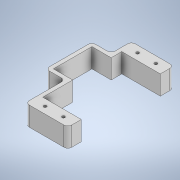
# Autodesk Inventor part: servo_bracket
Saved by Autodesk Inventor 2020 (Build 240168000, 168)
## iProperties
Created: 2019-05-08
Part Number: servo_bracket
Material: Generic
Document SubType Name: Modeling
Designer: erwin
Density: 1 g/cm^3
Appearance: Default
Author: erwin
Autodesk Inventor part; units mm, degrees
ref_plane "YZ Plane" through (0, 0, 0) normal (1, 0, 0) x (0, 1, 0)
ref_plane "XZ Plane" through (0, 0, 0) normal (0, 1, 0) x (-1, 0, 0)
ref_plane "XY Plane" through (0, 0, 0) normal (0, 0, 1) x (1, 0, 0)
sketch "Sketch1" plane through (0, 0, 0) normal (0, 1, 0) x (-1, 0, 0)
  line L0 (-9.6397, 29.7296) -> (10.3603, 29.7296)
  line L1 (12.3603, 29.7296) -> (12.3603, 36.7296)
  line L2 (12.3603, 36.7296) -> (-9.6397, 36.7296)
  line L3 (-9.6397, 36.7296) -> (-9.6397, 29.7296)
  line L4 (12.3603, 36.7296) -> (8.0662, 36.7296)
  line L5 (8.0662, -18.2704) -> (12.3603, -18.2704)
  line L6 (12.3603, -18.2704) -> (-9.6397, -18.2704)
  line L7 (-9.6397, -18.2704) -> (-9.6397, -11.2704)
  line L8 (-9.6397, -11.2704) -> (10.3603, -11.2704)
  line L9 (12.3603, -11.2704) -> (12.3603, -18.2704)
  line L10 (12.3603, -7.7704) -> (22.3603, -7.7704)
  line L11 (22.3603, -7.7704) -> (22.3603, 16.2296)
  line L12 (22.3603, 16.2296) -> (12.3603, 16.2296)
  line L13 (12.3603, -18.2704) -> (12.3603, -7.7704)
  line L14 (12.3603, 16.2296) -> (12.3603, 36.7296)
  line L15 (10.3603, 14.2296) -> (20.3603, 14.2296)
  line L16 (20.3603, 14.2296) -> (20.3603, -5.7704)
  line L17 (20.3603, -5.7704) -> (10.3603, -5.7704)
  line L18 (10.3603, 22.4354) -> (10.3603, 14.2296)
  line L19 (10.3603, -5.7704) -> (10.3603, -4.741)
  line L20 (10.3603, 29.7296) -> (10.3603, 14.2296)
  line L21 (10.3603, -5.7704) -> (10.3603, -11.2704)
  point P0 (0, 0)
  dimension "wall" = 2
  dimension "d1" = 2
  dimension "d2" = 2
  dimension "d3" = 2
  dimension "d4" = 2
  dimension "d5" = 7
  dimension "d6" = 7
  dimension "d7" = 20
  dimension "d8" = 20
  dimension "d9" = 41
  dimension "d10" = 5.5
  dimension "d11" = 20
  dimension "d12" = 10
  constraints: 44 end point, 13 parallel, 6 perpendicular, 5 horizontal, 2 point on line
  measures "wall" distance between parallel lines of L15 L12
  measures "d1" distance between parallel lines of L11 L16
  measures "d2" distance between parallel lines of L10 L17
  measures "d3" distance between parallel lines of L13 L21
  measures "d4" distance between parallel lines of L14 L20
  measures "d5" distance between parallel lines of L2 L0
  measures "d6" distance between parallel lines of L6 L8
  measures "d7" distance of L0.start L0.end
  measures "d8" distance of L7.end L8.end
  measures "d9" distance between parallel lines of L8 L0
  measures "d10" distance of L17.end L8.end
  measures "d11" distance of L15.end L16.end
  measures "d12" distance of L15.start L15.end
extrude "Extrusion1" add sketch "Sketch1" along normal blind 10
sketch "Sketch2" plane through (0, 10, 0) normal (0, 1, 0) x (1, 0, 0)
  line L0 (-10.3603, -29.7296) -> (-10.3603, -14.2296) construction
  line L1 (-12.3603, -36.7296) -> (9.6397, -36.7296) construction
  line L2 (9.6397, 18.2704) -> (-12.3603, 18.2704) construction
  line L3 (3.8669, 14.7392) -> (-5.6603, 14.7392) construction
  line L4 (-5.6603, 14.7392) -> (-5.6603, -33.2296) construction
  line L5 (-5.6603, -33.2296) -> (3.8669, -33.2296) construction
  line L6 (3.8669, -33.2296) -> (3.8669, 14.7392) construction
  point P0 (0, 0)
  point P1 (3.8397, -33.2296)
  point P2 (-5.6603, 14.7704)
  dimension "d15" = 4.7
  dimension "d16" = 9.5
  dimension "d17" = 48
  dimension "d18" = 3.5
  dimension "d19" = 3.5
  constraints: 8 end point, 2 parallel, 1 horizontal, 1 perpendicular
  measures "d15" distance from line of L0 L4.end
  measures "d16" distance of point (3.84, -33.23) L4.end
  measures "d17" distance of point (-5.66, 14.77) L4.end
  measures "d18" distance from line of L1 L4.end
  measures "d19" distance from line of L2 point (-5.66, 14.77)
hole "Hole1" at (-5.6603, 10, 33.2296) at (3.8397, 10, 33.2296) at (3.8669, 10, -14.7392) at (-5.6603, 10, -14.7704) direction (0, -1, 0) diameter 1.5 end through all
fillet "Fillet1" radius 2 8 edges at (9.6397, 5, 36.7296) (-12.3603, 5, 36.7296) (9.6397, 5, -18.2704) (-12.3603, 5, -18.2704) (-22.3603, 5, -7.7704) (-12.3603, 5, -7.7704) (-22.3603, 5, 16.2296) (-12.3603, 5, 16.2296)
equation "\"d1\" = wall"
equation "\"d2\" = wall"
equation "\"d3\" = wall"
equation "\"d4\" = wall"
equation "\"d6\" = d5"
equation "\"d8\" = d7"
equation "\"d19\" = d18"
body "Solid1"
